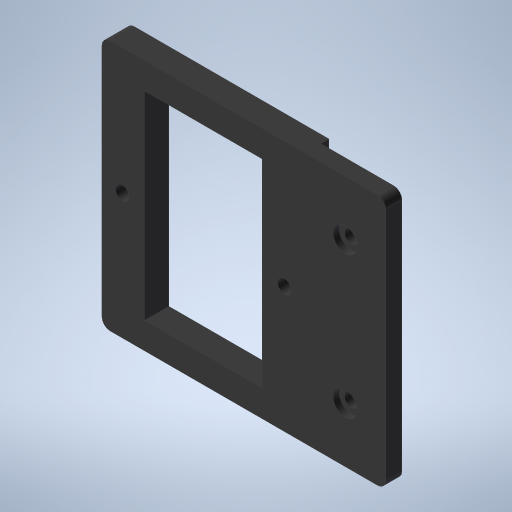
# Autodesk Inventor part: power_switch_bracket
Saved by Autodesk Inventor 2024.2 (Build 282272000, 272)
## iProperties
Created: 2024-06-03
Part Number: power_switch_bracket
Material: Generic
Document SubType Name: Modeling
Designer: Micha
Density: 1 g/cm^3
Appearance: Default
Author: Micha
Autodesk Inventor part; units mm, degrees
ref_plane "YZ Plane" through (0, 0, 0) normal (1, 0, 0) x (0, 1, 0)
ref_plane "XZ Plane" through (0, 0, 0) normal (0, 1, 0) x (-1, 0, 0)
ref_plane "XY Plane" through (0, 0, 0) normal (0, 0, 1) x (1, 0, 0)
sketch "Sketch1" plane through (0, 0, 0) normal (0, 0, 1) x (1, 0, 0)
  line L0 (0, 0) -> (50, 0)
  line L1 (50, 0) -> (50, 62)
  line L2 (50, 62) -> (0, 62)
  line L3 (0, 62) -> (0, 0)
  circle A0 centre (5, 31) radius 1.7
  circle A1 centre (45, 31) radius 1.7
  line L4 (10.5, 55.5) -> (39.5, 55.5)
  line L5 (39.5, 55.5) -> (39.5, 6.5)
  line L6 (39.5, 6.5) -> (10.5, 6.5)
  line L7 (10.5, 6.5) -> (10.5, 55.5)
  line L8 (25, 55.5) -> (25, 6.5) construction
  point P0 (10.5, 31)
  point P1 (39.5, 31)
  point P2 (50, 31)
  dimension "d0" = 3.4
  dimension "d1" = 3.4
  dimension "d2" = 40
  dimension "d3" = 29
  dimension "d4" = 49
  dimension "d5" = 5
  dimension "d6" = 5
  dimension "d7" = 62
  constraints: 18 end point, 5 midpoint, 4 parallel, 2 centre point, 2 horizontal, 2 horizontal alignment, 2 perpendicular, 1 symmetric about line
  measures "d0" diameter of A0
  measures "d1" diameter of A1
  measures "d2" distance of A1.centre A0.centre
  measures "d3" distance of L4.start L4.end
  measures "d4" distance of L4.end L5.end
  measures "d5" distance from line of L1 A1.centre
  measures "d6" distance from line of L3 A0.centre
  measures "d7" distance of L0.end L1.end
extrude "Extrusion1" add sketch "Sketch1" along normal blind 6
sketch "Sketch3" plane through (0, 0, 6) normal (0, 0, 1) x (1, 0, 0)
  line L0 (50, 62) -> (0, 62) projected
  line L1 (50, 62) -> (70, 62)
  line L2 (70, 62) -> (70, 0)
  line L3 (70, 0) -> (50, 0)
  line L4 (50, 0) -> (50, 62)
  circle A0 centre (60, 48.5) radius 1.7
  circle A1 centre (60, 13.5) radius 1.7
  line L5 (60, 48.5) -> (60, 13.5) construction
  point P0 (0, 0)
  point P1 (60, 0)
  point P2 (60, 31)
  point P3 (70, 31)
  dimension "d14" = 20
  dimension "d15" = 3.4
  dimension "d16" = 3.4
  dimension "d17" = 35
  constraints: 10 end point, 3 midpoint, 2 centre point, 2 parallel, 2 vertical alignment, 1 coincident, 1 horizontal, 1 horizontal alignment, 1 perpendicular, 1 vertical
  measures "d14" distance of L2.end L3.end
  measures "d15" diameter of A0
  measures "d16" diameter of A1
  measures "d17" distance of L5.end L5.start
extrude "Extrusion3" add sketch "Sketch3" against normal blind 4
sketch "Sketch4" plane through (0, 0, 6) normal (0, 0, 1) x (1, 0, 0)
  circle A0 centre (60, 48.5) radius 1.7 projected
  circle A1 centre (60, 13.5) radius 1.7 projected
  circle A2 centre (60, 48.5) radius 1.7 projected
  circle A3 centre (60, 48.5) radius 3
  circle A4 centre (60, 13.5) radius 1.7 projected
  circle A5 centre (60, 13.5) radius 3
  point P0 (0, 0)
  dimension "d20" = 6
  dimension "d21" = 6
  constraints: 2 centre point, 2 coincident
  measures "d20" diameter of A3
  measures "d21" diameter of A5
extrude "Extrusion4" cut sketch "Sketch4" against normal blind 1.5
fillet "Fillet1" radius 2 4 edges at (0, 62, 3) (0, 0, 3) (70, 0, 4) (70, 62, 4)
body "Solid1"
